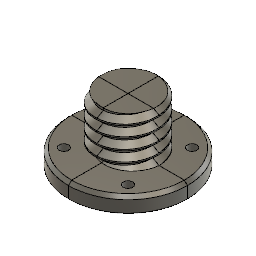
SideMount (Autodesk Fusion 360 design; units mm, degrees)
Autodesk Fusion 360 part; units mm, degrees
sketch "Sketch1" plane through (0, 0, 0) normal (0, 1, 0) x (1, 0, 0)
  circle A0 centre (0, 0) radius 20
  circle A1 centre (0, 0) radius 38.1
  line L0 (0, 0) -> (50, 0) construction
  line L1 (0, 0) -> (50, 0) construction
  line L2 (0, 0) -> (50, 0) construction
  line L3 (0, 0) -> (38.1, 0) construction
  line L4 (-26.9408, 26.9408) -> (-14.1421, 14.1421)
  line L5 (-20.5415, 20.5415) -> (20.5415, 20.5415)
  line L6 (20.5415, 20.5415) -> (20.5415, -20.5415)
  line L7 (20.5415, -20.5415) -> (-20.5415, -20.5415)
  line L8 (-20.5415, -20.5415) -> (-20.5415, 20.5415)
  line L9 (-20.5415, 20.5415) -> (20.5415, -20.5415) construction
  line L10 (20.5415, 20.5415) -> (-20.5415, -20.5415) construction
  dimension "d1" = 40
  dimension "d9" = 76.2
  measures "d1" diameter of A0
  measures "d9" diameter of A1
extrude "Extrude1" add sketch "Sketch1" along normal blind 30 contours A0 makes body 1
extrude "Extrude2" add sketch "Sketch1" against normal blind 10 contours A0 | A1 | L5 L6 L7 L8 bodies 1
chamfer "Chamfer1" distance 2 angle 45 1 edges at (-35.5217, 0, 13.7775) on bodies 1
chamfer "Chamfer2" distance 0.5 angle 45 1 edges at (-35.5217, -10, -13.7775) on bodies 1
thread "Thread2" "ISO Metric Trapezoidal Threads 40.0 TR40x7 7e" major diameter 39.7875 minor diameter 31.7155 pitch 7 angle 60 modelled right hand crest width 0.875 on face at (19.9006, 10, 1.9914) crest through (19.8938, -0.4375, 0) on bodies 1
hole "Hole1" at (-20.5415, 0, -20.5415) at (20.5415, 0, -20.5415) at (20.5415, 0, 20.5415) at (-20.5415, 0, 20.5415) direction (0, -1, 0) diameter 6.0452 depth 21 tip angle 118 bodies 1
extrude "Extrude3" add sketch "Sketch1" along normal blind -31.904 and the other way blind 15.719 separate body contours A0 | L5 L6 L7 L8 makes body 2
ref_plane "WorkPlane1" through (0, -23.8115, 0) normal (0, 0, 1) x (-1, 0, 0)
ref_plane "WorkPlane2" through (0, -23.8115, 0) normal (-1, 0, 0) x (0, 0, -1)
split "Split1" by plane through (0, -23.8115, 0) normal (-1, 0, 0) bodies 1 makes body 3 at (-5.9746, -10, 6.3434)
split "Split2" by plane through (0, -23.8115, 0) normal (0, 0, 1) bodies 1 3 makes body 5 at (-19.2303, -10, 5.8509) makes body 4 at (19.2303, -10, 5.8509)
hidden bodies 2
equation "d9 = 38.10 mm * 2"
equation "d14 = 0.138 in + 0.1 in"
named bodies: "TileScrewMountBody", "MidplaneBody", "TileScrewMountBody (1)", "TileScrewMountBody (2)", "TileScrewMountBody (1) (1)"
